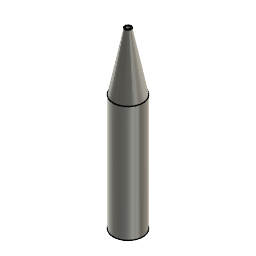
Pull Hook Assembly (Autodesk Fusion 360 archive; units mm, degrees)
design "Wire holder"
part number: 2026-07-29-12-23-19-486
Autodesk Fusion 360 part; units mm, degrees
sketch "Sketch1" plane through (0, 0, 0) normal (0, 0, 1) x (1, 0, 0)
  circle A0 centre (0, 0) radius 0.35
  circle A1 centre (0, 0) radius 2.545
  dimension "d1" = 0.7
  dimension "d2" = 5.09
  constraint coincident A0.centre A1.centre
  constraint concentric A0 A1
  measures "d1" diameter of A0
  measures "d2" diameter of A1
extrude "Extrude1" add sketch "Sketch1" along normal blind 30
chamfer "Chamfer1" distance 2 distance2 10 1 edges at (-2.3728, -0.9203, 30) measured on face at (1.8039, -0.1264, 30)

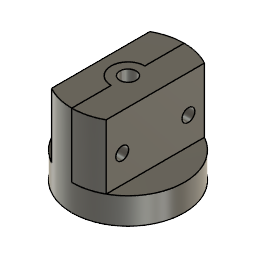
design "Hook mount Final"
part number: 2026-07-02-00-52-41-299
Autodesk Fusion 360 part; units mm, degrees
sketch "Sketch1" plane through (0, 0, 0) normal (0, 0, 1) x (1, 0, 0)
  circle A0 centre (0, 0) radius 17.5
  dimension "d1" = 35
  constraint coincident A0.centre origin
  measures "d1" diameter of A0
extrude "Extrude1" add sketch "Sketch1" along normal blind 8.2 makes body 1
sketch "Sketch2" plane through (0, 0, 8.2) normal (0, 0, 1) x (-1, 0, 0)
  circle A0 centre (0, 0) radius 17.5
  circle A1 centre (0, 0) radius 3
  dimension "d4" = 6
  constraint coincident A0.centre A1.centre
  measures "d4" diameter of A1
extrude "Extrude2" cut sketch "Sketch2" against normal through all contours A1 bodies 1
sketch "Sketch3" plane through (0, 0, 8.2) normal (0, 0, 1) x (-1, 0, 0)
  circle A0 centre (0, 0) radius 3
  circle A1 centre (0, 0) radius 17.5
  circle A2 centre (0, 0) radius 5.25
  dimension "d7" = 10.5
  constraint coincident A0.centre A1.centre
  measures "d7" diameter of A2
extrude "Extrude3" cut sketch "Sketch3" against normal blind 6.2 contours A2 bodies 1
sketch "Sketch4" plane through (0, 0, 8.2) normal (0, 0, 1) x (-1, 0, 0)
  circle A0 centre (0, 0) radius 5.25
  circle A1 centre (0, 0) radius 17.5
  line L0 (0, -17.5) -> (0, 17.5)
  circle A2 centre (0, 0) radius 17.5
  circle A3 centre (0, 0) radius 17.5
  constraint coincident A1 L0.start
  constraint coincident A1 L0.end
  constraint vertical L0
  constraint coincident L0 A0.centre
  constraint coincident A0.centre A1.centre
  constraint equal A2 A3
extrude "Extrude4" add sketch "Sketch4" along normal blind 20 contours A0 A1 L0 A2 A3 picked at (13.3573, -0.8302) bodies 1
sketch "Sketch5" plane through (0, 0, 8.2) normal (0, 0, 1) x (-1, 0, 0)
  line L0 (0, -17.5) -> (0, -5.25)
  arc A0 (0, 5.25) -> (0, -5.25) centre (0, 0) ccw
  line L1 (0, 5.25) -> (0, 17.5)
  arc A1 (0, 17.5) -> (0, -17.5) centre (0, 0) ccw
  circle A2 centre (0, 0) radius 5.25
  dimension "d12" = 10.5
  constraint coincident A0.centre A1.centre
  measures "d12" diameter of A2
extrude "Extrude5" add sketch "Sketch5" along normal up to surface (20 mm away) separate body makes body 2
sketch "Sketch6" plane through (0, 0, 28.2) normal (0, 0, 1) x (-1, 0, 0)
  line L0 (0, 17.5) -> (0, 5.25)
  arc A0 (0, -5.25) -> (0, 5.25) centre (0, 0) ccw
  line L1 (0, -5.25) -> (0, -17.5)
  arc A1 (0, -17.5) -> (0, 17.5) centre (0, 0) ccw
sketch "Sketch11" plane through (0, 0, 28.2) normal (0, 0, 1) x (-1, 0, 0)
  arc A0 (5.2262, 0.4994) -> (5.2262, -0.4994) centre (5.25, 0) ccw
  arc A1 (5.2262, 0.4994) -> (0, 5.25) centre (0, 0) ccw
  line L0 (0, 5.25) -> (0, 17.5)
  arc A2 (0, 17.5) -> (0, -17.5) centre (0, 0) ccw
  line L1 (0, -17.5) -> (0, -5.25)
  arc A3 (0, -5.25) -> (5.2262, -0.4994) centre (0, 0) ccw
  line L2 (-8.5, -15.2971) -> (-8.5, 15.2971)
  line L3 (8.5, -15.2971) -> (8.5, 15.2971)
  arc A4 (0, -17.5) -> (0, 17.5) centre (0, 0) ccw
  dimension "d35" = 17
  dimension "d36" = 8.5
  constraint coincident A2 L2.start
  constraint coincident A2 L2.end
  constraint vertical L2
  constraint parallel L0 L3
  constraint coincident L3.start A4
  constraint coincident L3.end A4
  measures "d35" distance of L2 L3
  measures "d36" distance of L1 L3
extrude "Extrude10" cut sketch "Sketch11" against normal blind 20 contours A2 L2 | L3 A4 bodies 1 2
sketch "Sketch7" plane through (8.5, 0, 0) normal (1, 0, 0) x (0, 1, 0)
  line L0 (-17.5, 16.7) -> (17.5, 16.7) construction
  line L1 (17.5, 8.2) -> (17.5, 28.2)
  line L2 (-17.5, 8.2) -> (-17.5, 28.2)
  circle A0 centre (-10.2971, 16.7) radius 2
  circle A1 centre (10.2971, 16.7) radius 2
  line L3 (15.2971, 28.2) -> (-15.2971, 28.2)
  line L4 (-15.2971, 28.2) -> (-15.2971, 8.2)
  line L5 (-15.2971, 8.2) -> (15.2971, 8.2)
  line L6 (15.2971, 8.2) -> (15.2971, 28.2)
  dimension "d20" = 8.5
  dimension "d21" = 4
  dimension "d39" = 5
  dimension "d40" = 5
  constraint horizontal L0
  constraint coincident L0.end L1
  constraint coincident L0.start L2
  constraint coincident L0 A0.centre
  constraint coincident L0 A1.centre
  constraint equal A0 A1
  measures "d20" distance of L0 L2.start
  measures "d21" diameter of A1
  measures "d39" distance of A0.centre L4
  measures "d40" distance of A1.centre L6
extrude "Extrude6" cut sketch "Sketch7" against normal blind 8.5 contours A0 | A1 bodies 2
sketch "Sketch10" plane through (0, 0, 28.2) normal (0, 0, 1) x (-1, 0, 0)
  line L0 (0, -17.5) -> (0, -5.25)
  arc A0 (0, -5.25) -> (0, 5.25) centre (0, 0) ccw
  line L1 (0, 5.25) -> (0, 17.5)
  circle A1 centre (0, 0) radius 2.55
  arc A2 (-8.5, -15.2971) -> (0, -17.5) centre (0, 0) ccw
  line L2 (-8.5, 15.2971) -> (-8.5, -15.2971)
  arc A3 (0, 17.5) -> (-8.5, 15.2971) centre (0, 0) ccw
  dimension "d32" = 5.1
  constraint coincident A0.centre A1.centre
  measures "d32" diameter of A1
extrude "Extrude9" cut sketch "Sketch10" against normal blind 10 contours A1 bodies 2
sketch "Sketch12" plane through (-8.5, 0, 0) normal (-1, 0, 0) x (0, -1, 0)
  line L0 (15.2971, 28.2) -> (-15.2971, 28.2)
  line L1 (-15.2971, 28.2) -> (-15.2971, 8.2)
  line L2 (-15.2971, 8.2) -> (15.2971, 8.2)
  line L3 (15.2971, 8.2) -> (15.2971, 28.2)
  circle A0 centre (-10.2971, 16.7) radius 2.05
  circle A1 centre (10.2971, 16.7) radius 2.05
  point P0 (-10.2971, 16.7)
  point P1 (10.2971, 16.7)
  dimension "d42" = 4.1
  constraint coincident P0 A0.centre
  constraint coincident P1 A1.centre
  constraint equal A0 A1
  measures "d42" diameter of A0
extrude "Extrude11" cut sketch "Sketch12" against normal blind 8.5 contours A0 | A1 bodies 1
named bodies: "Body A", "Body B"
